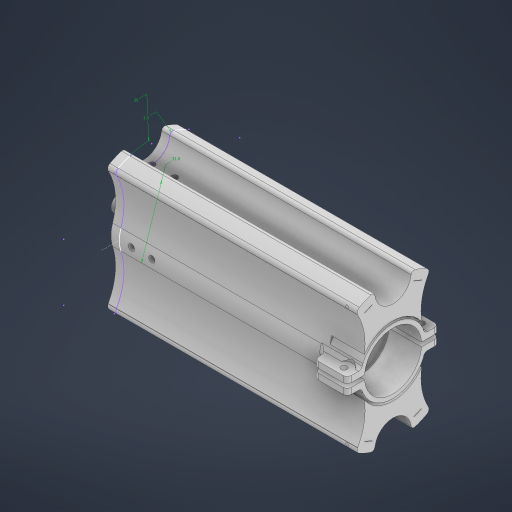
# Autodesk Inventor part: michigandrummy
Saved by Autodesk Inventor 2024.2 (Build 282272000, 272)
## iProperties
Created: 2024-04-03
Part Number: michigandrummy
Material: Generic
Document SubType Name: Modeling
Designer: jerem
Density: 1 g/cm^3
Appearance: Default
Author: jerem
## iProperties of the stored document michigandrummy_3DPrint.ipt
Created: 2024-04-05
Part Number: michigandrummy_3DPrint
Material: Generic
Document SubType Name: Modeling
Designer: jerem
Density: 1 g/cm^3
Appearance: Default
Author: jerem
Autodesk Inventor part; units mm, degrees
ref_plane "YZ Plane" through (0, 0, 0) normal (1, 0, 0) x (0, 1, 0)
ref_plane "XZ Plane" through (0, 0, 0) normal (0, 1, 0) x (-1, 0, 0)
ref_plane "XY Plane" through (0, 0, 0) normal (0, 0, 1) x (1, 0, 0)
sketch "Sketch1" plane through (0, 0, 0) normal (1, 0, 0) x (0, 1, 0)
  arc A0 (1, -13.864) -> (1, 13.864) centre (0, 0) ccw
  line L0 (0, 0) -> (1, 0) construction
  line L1 (1, 13.864) -> (1, 22.3886)
  line L2 (1, 22.3886) -> (4, 22.3886)
  line L3 (4, 22.3886) -> (4, 15.3886)
  line L4 (1, -13.864) -> (1, -22.3886)
  line L5 (1, -22.3886) -> (4, -22.3886)
  line L6 (4, -22.3886) -> (4, -15.3886)
  arc A1 (4, -15.3886) -> (4, 15.3886) centre (0, 0) ccw
  point P0 (4, -15.3886)
  point P1 (4, 15.3886)
  dimension "d0" = 27.8
  dimension "d1" = 1
  dimension "d3" = 3
  dimension "d4" = 2
  dimension "d5" = 1
  dimension "d11" = 7
  constraints: 14 end point, 4 point on circle, 2 centre point, 2 coincident, 2 collinear, 2 horizontal, 2 symmetric about line, 1 perpendicular, 1 vertical
  measures "d0" diameter of A0
  measures "d1" distance of L0.start L0.end
  measures "d3" distance of L1.end L2.end
  measures "d4" radial gap between concentric circles of A0 A1
  measures "d5" distance from line of point (0, 0) L1
  measures "d11" distance of L3.end L2.end
extrude "Extrusion1" add sketch "Sketch1" along normal blind 16
sketch "Sketch2" plane through (0, 4, 22.3886) normal (0, 1, 0) x (1, 0, 0)
  line L0 (0, 7) -> (16, 7) construction
  line L1 (16, 0) -> (16, 8.5247) construction
  line L2 (16, 7) -> (16, 0) construction
  circle A0 centre (11, 3.5) radius 1.5
  line L3 (16, 36.2526) -> (16, 8.5247) projected
  line L4 (16, 22.3886) -> (0, 22.3886)
  circle A1 centre (11, 41.2773) radius 1.5
  line L5 (11, 41.2773) -> (11, 37.7773) construction
  line L6 (0, 37.7773) -> (16, 37.7773) construction
  line L7 (11, 3.5) -> (11, 7) construction
  point P0 (16, 3.5)
  dimension "d8" = 5
  dimension "d9" = 3
  dimension "d10" = 3.5
  constraints: 8 end point, 3 point on line, 2 centre point, 2 midpoint, 1 collinear, 1 horizontal, 1 symmetric about line, 1 vertical, 1 other
  measures "d8" distance of point (16, 3.5) L7.start
  measures "d9" diameter of A0
  measures "d10" distance of L7.start L7.end
extrude "Extrusion2" cut sketch "Sketch2" along normal through all both and the other way through all
mirror "Mirror1" about plane through (0, 0, 0) normal (0, 1, 0) of "Extrusion1", "Extrusion2"
fillet "Fillet1" radius 2 4 edges at (8, 4, 15.3886) (8, -4, 15.3886) (8, 4, -15.3886) (8, -4, -15.3886)
sketch "Sketch3" plane through (0, -4, -22.3886) normal (-1, 0, 0) x (0, 0, 1)
  circle A0 centre (22.3886, 4) radius 13.9
  circle A1 centre (22.3886, 4) radius 15.9
  circle A2 centre (22.3886, 4) radius 4.85
  dimension "d15" = 9.7
  dimension "d19" = 27.8
  dimension "d20" = 2
  constraints: 3 centre point, 3 coincident
  measures "d15" diameter of A2
  measures "d19" diameter of A0
  measures "d20" radial gap between concentric circles of A0 A1
extrude "Extrusion3" add sketch "Sketch3" along normal blind 4.2 contours A0 | A1
sketch "Sketch4" plane through (-4.2, 0, 0) normal (-1, 0, 0) x (0, 0, 1)
  circle A0 centre (0, 0) radius 4.85
  circle A1 centre (0, 0) radius 15.9
  circle A2 centre (0, 0) radius 4.85 projected
  circle A3 centre (0, 0) radius 1.5
  dimension "d18" = 3
  dimension "d21" = 31.8
  constraints: 3 centre point, 2 coincident
  measures "d18" diameter of A3
  measures "d21" diameter of A1
extrude "Extrusion4" add sketch "Sketch4" along normal blind 10 contours A0 | A1
fillet "Fillet2" radius 4 4 edges at (0, -3.1958, 15.5755) (0, 3.1958, 15.5755) (0, -3.1958, -15.5755) (0, 3.1958, -15.5755)
sketch "Sketch5" plane through (-14.2, 0, 0) normal (-1, 0, 0) x (0, 0, 1)
  circle A0 centre (0, 0) radius 1.5 projected
  circle A1 centre (0, 0) radius 2
  circle A2 centre (0, 0) radius 4
  dimension "d25" = 4
  dimension "d26" = 2
  constraints: 2 centre point, 2 coincident
  measures "d25" diameter of A1
  measures "d26" radial gap between concentric circles of A1 A2
extrude "Extrusion5" add sketch "Sketch5" along normal blind 87.8 contours A2
sketch "Sketch6" plane through (0, 0, 0) normal (1, 0, 0) x (0, 1, 0)
  circle A0 centre (0, 0) radius 1.5 construction
  circle A1 centre (0, 0) radius 35 construction
  line L0 (35, 0) -> (25, 0)
  line L1 (31.6536, -14.9349) -> (22.6097, -10.6678)
  arc A2 (31.6536, -14.9349) -> (35, 0) centre (0, 0) ccw construction
  dimension "d29" = 70
  dimension "d30" = 10
  dimension "d31" = 10
  constraints: 4 end point, 4 point on circle, 2 centre point, 1 coincident, 1 concentric, 1 horizontal, 1 line through centre
  measures "d29" diameter of A1
  measures "d30" distance of L0.start L0.end
  measures "d31" distance of L1.start L1.end
sketch "Sketch7" plane through (-102, 0, 0) normal (-1, 0, 0) x (0, 0, 1)
  circle A0 centre (0, 0) radius 15.9
  circle A1 centre (0, 0) radius 1.5 projected
  line L0 (0, 0) -> (24.7477, 0) construction
  line L1 (-24.9082, 0) -> (-15.9, 0)
  line L2 (-1.5, 0) -> (15.9, 0)
  line L3 (17.3493, 28.2476) -> (17.2713, 28.1124)
  line L4 (0.1605, 0) -> (15.9, 0)
  arc A2 (0, 24.1323) -> (8.826, 31.8269) centre (0, 33.0415) ccw
  arc A3 (17.3493, 28.2476) -> (15.119, 4.9221) centre (43.0631, 14.0195) ccw
  arc A4 (0, 24.1323) -> (8.852, 32.0333) centre (0, 33.0415) ccw
  arc A5 (16.481, 30.8768) -> (10.8054, 33.2903) centre (0, 0) ccw
  line L5 (0, 15.9) -> (0, 24.1323)
  line L6 (-17.3493, 28.2476) -> (-17.2713, 28.1124)
  arc A6 (-15.119, 4.9221) -> (-17.3493, 28.2476) centre (-43.0631, 14.0195) ccw
  arc A7 (-8.852, 32.0333) -> (0, 24.1323) centre (0, 33.0415) ccw
  arc A8 (-10.8054, 33.2903) -> (-16.481, 30.8768) centre (0, 0) ccw
  arc A9 (-16.481, 30.8768) -> (-17.2713, 28.1124) centre (-15.5392, 29.1124) ccw
  arc A10 (17.2713, 28.1124) -> (16.481, 30.8768) centre (15.5392, 29.1124) ccw
  arc A11 (-8.852, 32.0333) -> (-10.8054, 33.2903) centre (-10.3423, 31.8636) ccw
  arc A12 (10.8054, 33.2903) -> (8.852, 32.0333) centre (10.3423, 31.8636) ccw
  line L7 (17.3493, -28.2476) -> (17.2713, -28.1124)
  arc A13 (8.826, -31.8269) -> (0, -24.1323) centre (0, -33.0415) ccw
  arc A14 (15.119, -4.9221) -> (17.3493, -28.2476) centre (43.0631, -14.0195) ccw
  arc A15 (8.852, -32.0333) -> (0, -24.1323) centre (0, -33.0415) ccw
  arc A16 (10.8054, -33.2903) -> (16.481, -30.8768) centre (0, 0) ccw
  line L8 (0, -15.9) -> (0, -24.1323)
  arc A17 (-16.481, -30.8768) -> (-10.8054, -33.2903) centre (0, 0) ccw
  arc A18 (-17.3493, -28.2476) -> (-15.119, -4.9221) centre (-43.0631, -14.0195) ccw
  line L9 (-17.3493, -28.2476) -> (-17.2713, -28.1124)
  arc A19 (0, -24.1323) -> (-8.852, -32.0333) centre (0, -33.0415) ccw
  arc A20 (-17.2713, -28.1124) -> (-16.481, -30.8768) centre (-15.5392, -29.1124) ccw
  arc A21 (16.481, -30.8768) -> (17.2713, -28.1124) centre (15.5392, -29.1124) ccw
  arc A22 (-10.8054, -33.2903) -> (-8.852, -32.0333) centre (-10.3423, -31.8636) ccw
  arc A23 (8.852, -32.0333) -> (10.8054, -33.2903) centre (10.3423, -31.8636) ccw
  point P0 (18.2746, 29.8503)
  point P1 (-8.826, 31.8269)
  point P2 (-18.2746, 29.8503)
  point P3 (18.2746, -29.8503)
  point P4 (-8.826, -31.8269)
  point P5 (-18.2746, -29.8503)
  point P6 (8.826, 31.8269)
  point P7 (-15.119, 4.9221)
  point P8 (-15.119, -4.9221)
  point P9 (15.119, -4.9221)
  dimension "d36" = 35
  dimension "d40" = 1.5
  dimension "d41" = 31.8
  constraints: 54 point on circle, 30 symmetric about line, 23 centre point, 20 end point, 9 tangent, 6 point on line, 4 coincident, 2 equal radius, 1 horizontal, 1 horizontal alignment, 15 other
  measures "d36" radius of A5
  measures "d40" radius of A11
  measures "d41" diameter of A0
extrude "Extrusion6" add sketch "Sketch7" against normal up to surface (87.8 mm away)
sketch "Sketch8" plane through (-14.2, 0, 0) normal (1, 0, 0) x (0, 0, -1)
  circle A0 centre (0, 0) radius 35
  circle A1 centre (0, 0) radius 15.9
  arc A2 (-17.3493, -28.2476) -> (-15.119, -4.9221) centre (-43.0631, -14.0195) ccw projected
  arc A3 (15.119, 4.9221) -> (-15.119, 4.9221) centre (0, 0) ccw projected
  arc A4 (17.3493, 28.2476) -> (15.119, 4.9221) centre (43.0631, 14.0195) ccw projected
  line L0 (17.3493, 28.2476) -> (17.2713, 28.1124) projected
  arc A5 (17.2713, 28.1124) -> (16.481, 30.8768) centre (15.5392, 29.1124) ccw projected
  arc A6 (16.481, 30.8768) -> (10.8054, 33.2903) centre (0, 0) ccw projected
  arc A7 (10.8054, 33.2903) -> (8.852, 32.0333) centre (10.3423, 31.8636) ccw projected
  arc A8 (-8.852, 32.0333) -> (8.852, 32.0333) centre (0, 33.0415) ccw projected
  arc A9 (-8.852, 32.0333) -> (-10.8054, 33.2903) centre (-10.3423, 31.8636) ccw projected
  arc A10 (-10.8054, 33.2903) -> (-16.481, 30.8768) centre (0, 0) ccw projected
  arc A11 (-16.481, 30.8768) -> (-17.2713, 28.1124) centre (-15.5392, 29.1124) ccw projected
  line L1 (-17.2713, 28.1124) -> (-17.3493, 28.2476) projected
  arc A12 (-15.119, 4.9221) -> (-17.3493, 28.2476) centre (-43.0631, 14.0195) ccw projected
  arc A13 (-15.119, -4.9221) -> (15.119, -4.9221) centre (0, 0) ccw projected
  arc A14 (-17.3493, -28.2476) -> (-15.119, -4.9221) centre (-43.0631, -14.0195) ccw projected
  line L2 (-17.3493, -28.2476) -> (-17.2713, -28.1124) projected
  arc A15 (-17.2713, -28.1124) -> (-16.481, -30.8768) centre (-15.5392, -29.1124) ccw projected
  arc A16 (-16.481, -30.8768) -> (-10.8054, -33.2903) centre (0, 0) ccw projected
  arc A17 (-10.8054, -33.2903) -> (-8.852, -32.0333) centre (-10.3423, -31.8636) ccw projected
  arc A18 (8.852, -32.0333) -> (-8.852, -32.0333) centre (0, -33.0415) ccw projected
  arc A19 (8.852, -32.0333) -> (10.8054, -33.2903) centre (10.3423, -31.8636) ccw projected
  arc A20 (10.8054, -33.2903) -> (16.481, -30.8768) centre (0, 0) ccw projected
  arc A21 (16.481, -30.8768) -> (17.2713, -28.1124) centre (15.5392, -29.1124) ccw projected
  line L3 (17.2713, -28.1124) -> (17.3493, -28.2476) projected
  arc A22 (15.119, -4.9221) -> (17.3493, -28.2476) centre (43.0631, -14.0195) ccw projected
  point P0 (16.481, 30.8768)
  point P1 (10.8054, 33.2903)
  point P2 (-10.8054, 33.2903)
  point P3 (-16.481, 30.8768)
  point P4 (15.119, 4.9221)
  point P5 (-17.3493, -28.2476)
  point P6 (-16.481, -30.8768)
  point P7 (-10.8054, -33.2903)
  point P8 (10.8054, -33.2903)
  point P9 (16.481, -30.8768)
  point P10 (15.119, -4.9221)
  dimension "d44" = 70
  constraints: 2 coincident, 1 centre point, 2 other
  measures "d44" diameter of A0
extrude "Extrusion7" add sketch "Sketch8" along normal up to surface (30.2 mm away) contours A5 L0 A4 A1 A12 L1 A11 A0 A9 A8 A7 | A0 A19 A18 A17 A15 L2 A2 A1 A22 L3 A21
sketch "Sketch10" plane through (0, 4, 22.3886) normal (0, 1, 0) x (1, 0, 0)
  circle A0 centre (11, 3.5) radius 1.5 projected
  circle A1 centre (11, 41.2773) radius 1.5 projected
  circle A2 centre (11, 3.5) radius 1.5
  circle A3 centre (11, 41.2773) radius 1.5
  point P0 (0, 22.3886)
  point P1 (12.8189, 5.5242)
  point P2 (9.3832, 5.5242)
  point P3 (9.3832, 39.2531)
  point P4 (12.8189, 39.2531)
  point P5 (9.7518, 39.7146)
  point P6 (12.5, 41.2773)
  point P7 (12.3368, 4.9876)
  point P8 (12.5, 3.5)
  constraints: 2 centre point, 2 coincident, 4 other
extrude "Extrusion8" cut sketch "Sketch10" along normal mid plane 147.627
sketch "Sketch12" plane through (16, 0, 0) normal (1, 0, 0) x (0, 0, -1)
  arc A0 (17.3493, 28.2476) -> (15.0262, 5.212) centre (43.0631, 14.0195) ccw projected
  line L0 (17.2713, 28.1124) -> (17.3493, 28.2476) projected
  arc A1 (17.2713, 28.1124) -> (16.481, 30.8768) centre (15.5392, 29.1124) ccw projected
  arc A2 (16.481, 30.8768) -> (10.8054, 33.2903) centre (0, 0) ccw projected
  arc A3 (10.8054, 33.2903) -> (8.852, 32.0333) centre (10.3423, 31.8636) ccw projected
  arc A4 (-8.852, 32.0333) -> (8.852, 32.0333) centre (0, 33.0415) ccw projected
  arc A5 (-8.852, 32.0333) -> (-10.8054, 33.2903) centre (-10.3423, 31.8636) ccw projected
  arc A6 (-10.8054, 33.2903) -> (-16.481, 30.8768) centre (0, 0) ccw projected
  arc A7 (-16.481, 30.8768) -> (-17.2713, 28.1124) centre (-15.5392, 29.1124) ccw projected
  line L1 (-17.3493, 28.2476) -> (-17.2713, 28.1124) projected
  arc A8 (-15.0262, 5.212) -> (-17.3493, 28.2476) centre (-43.0631, 14.0195) ccw projected
  arc A9 (-16.8645, 4) -> (-15.0262, 5.212) centre (-16.8645, 6) ccw projected
  line L2 (-16.8645, 4) -> (-22.3886, 4) projected
  line L3 (-22.3886, 4) -> (-22.3886, 1) projected
  line L4 (-22.3886, 1) -> (-13.864, 1) projected
  arc A10 (13.864, 1) -> (-13.864, 1) centre (0, 0) ccw projected
  line L5 (13.864, 1) -> (22.3886, 1) projected
  line L6 (22.3886, 1) -> (22.3886, 4) projected
  line L7 (22.3886, 4) -> (16.8645, 4) projected
  arc A11 (15.0262, 5.212) -> (16.8645, 4) centre (16.8645, 6) ccw projected
  line L8 (-13.9332, 27.3327) -> (-10.2755, 28.8831)
  line L9 (-10.2755, 28.8831) -> (-10.1975, 28.6989)
  line L10 (-10.1975, 28.6989) -> (-13.8551, 27.1485)
  line L11 (-13.8551, 27.1485) -> (-13.9332, 27.3327)
  line L12 (-14.2092, 31.9859) -> (-14.2092, 31.9859)
  point P0 (-17.3103, 28.18)
  point P1 (-13.8941, 27.2406)
  point P2 (-10.2365, 28.791)
  point P3 (-12.1043, 28.1079)
  dimension "d63" = 0.2
  constraints: 10 end point, 4 midpoint, 3 perpendicular, 2 point on circle, 1 tangent
  measures "d63" distance from line of L10 point (-12.104, 28.108)
extrude "Extrusion10" cut sketch "Sketch12" against normal through all contours L8 L9 L10 L11
mirror "Mirror4" about plane through (0, 0, 0) normal (0, 1, 0) of "Extrusion10"
mirror "Mirror5" about plane through (0, 0, 0) normal (0, 0, 1) of "Extrusion10", "Mirror4"
extrude "Extrusion12" add sketch "Sketch7" along normal blind 4
sketch "Sketch13" plane through (-102, 0, 0) normal (-1, 0, 0) x (0, 0, 1)
  circle A0 centre (0, 0) radius 3.925
  circle A1 centre (0, 0) radius 1.5 projected
  circle A2 centre (0, 0) radius 1.5
  dimension "d64" = 7.85
  dimension "d65" = 3
  constraints: 2 centre point, 2 coincident
  measures "d64" diameter of A0
  measures "d65" diameter of A2
extrude "Extrusion11" add sketch "Sketch13" along normal blind 12 from surface at 4
sketch "Sketch14" plane through (-106, 0, 0) normal (-1, 0, 0) x (0, 0, 1)
  circle A0 centre (0, 0) radius 4.445
  circle A1 centre (0, 0) radius 2
  dimension "d70" = 8.89
  constraints: 2 centre point, 2 coincident
  measures "d70" diameter of A0
extrude "Extrusion13" add sketch "Sketch14" along normal blind 2 contours A0 | A1
sketch "Sketch15" plane through (16, 0, 0) normal (1, 0, 0) x (0, 0, -1)
  circle A0 centre (0, 0) radius 14
  dimension "d73" = 28
  constraints: 1 centre point, 1 coincident
  measures "d73" diameter of A0
extrude "Extrusion14" cut sketch "Sketch15" against normal up to surface (16 mm away)
sketch "Sketch16" plane through (0, 4, 22.3886) normal (0, 1, 0) x (1, 0, 0)
  circle A0 centre (11, 3.5) radius 1.5 projected
  circle A1 centre (11, 3.5) radius 4
  point P0 (0, 22.3886)
  dimension "d76" = 8
  constraints: 1 centre point, 1 coincident
  measures "d76" diameter of A1
extrude "Extrusion15" cut sketch "Sketch16" along normal blind 10
mirror "Mirror6" about plane through (0, 0, 0) normal (0, 1, 0) of "Extrusion15"
mirror "Mirror7" about plane through (0, 0, 0) normal (0, 0, 1) of "Extrusion15", "Mirror6"
sketch "Sketch17" plane through (16, 0, 0) normal (1, 0, 0) x (0, 0, -1)
  circle A0 centre (0, 0) radius 4.85 projected
  circle A1 centre (0, 0) radius 16
  circle A2 centre (0, 0) radius 1.5 projected
  circle A3 centre (0, 0) radius 17
  arc A4 (13.9642, 1) -> (-13.9642, 1) centre (0, 0) ccw projected
  line L0 (13.9642, 1) -> (22.3886, 1) projected
  line L1 (22.3886, 1) -> (22.3886, 4) projected
  line L2 (22.3886, 4) -> (16.8645, 4) projected
  arc A5 (15.0262, 5.212) -> (16.8645, 4) centre (16.8645, 6) ccw projected
  arc A6 (17.3493, 28.2476) -> (15.0262, 5.212) centre (43.0631, 14.0195) ccw projected
  line L3 (17.2713, 28.1124) -> (17.3493, 28.2476) projected
  arc A7 (17.2713, 28.1124) -> (16.481, 30.8768) centre (15.5392, 29.1124) ccw projected
  arc A8 (16.481, 30.8768) -> (10.8054, 33.2903) centre (0, 0) ccw projected
  arc A9 (10.8054, 33.2903) -> (8.852, 32.0333) centre (10.3423, 31.8636) ccw projected
  arc A10 (-8.852, 32.0333) -> (8.852, 32.0333) centre (0, 33.0415) ccw projected
  arc A11 (-8.852, 32.0333) -> (-10.8054, 33.2903) centre (-10.3423, 31.8636) ccw projected
  arc A12 (-10.8054, 33.2903) -> (-16.481, 30.8768) centre (0, 0) ccw projected
  arc A13 (-16.481, 30.8768) -> (-17.2713, 28.1124) centre (-15.5392, 29.1124) ccw projected
  line L4 (-17.3493, 28.2476) -> (-17.2713, 28.1124) projected
  arc A14 (-15.0262, 5.212) -> (-17.3493, 28.2476) centre (-43.0631, 14.0195) ccw projected
  arc A15 (-16.8645, 4) -> (-15.0262, 5.212) centre (-16.8645, 6) ccw projected
  line L5 (-16.8645, 4) -> (-22.3886, 4) projected
  line L6 (-22.3886, 4) -> (-22.3886, 1) projected
  line L7 (-22.3886, 1) -> (-13.9642, 1) projected
  line L8 (13.9332, 27.3327) -> (13.8551, 27.1485) projected
  line L9 (13.8551, 27.1485) -> (10.1975, 28.6989) projected
  line L10 (10.1975, 28.6989) -> (10.2755, 28.8831) projected
  line L11 (10.2755, 28.8831) -> (13.9332, 27.3327) projected
  line L12 (-10.2755, 28.8831) -> (-10.1975, 28.6989) projected
  line L13 (-10.1975, 28.6989) -> (-13.8551, 27.1485) projected
  line L14 (-13.8551, 27.1485) -> (-13.9332, 27.3327) projected
  line L15 (-13.9332, 27.3327) -> (-10.2755, 28.8831) projected
  arc A16 (-13.9642, -1) -> (13.9642, -1) centre (0, 0) ccw projected
  line L16 (-22.3886, -1) -> (-13.9642, -1) projected
  line L17 (-22.3886, -4) -> (-22.3886, -1) projected
  line L18 (-16.8645, -4) -> (-22.3886, -4) projected
  arc A17 (-15.0262, -5.212) -> (-16.8645, -4) centre (-16.8645, -6) ccw projected
  arc A18 (-17.3493, -28.2476) -> (-15.0262, -5.212) centre (-43.0631, -14.0195) ccw projected
  line L19 (-17.2713, -28.1124) -> (-17.3493, -28.2476) projected
  arc A19 (-17.2713, -28.1124) -> (-16.481, -30.8768) centre (-15.5392, -29.1124) ccw projected
  arc A20 (-16.481, -30.8768) -> (-10.8054, -33.2903) centre (0, 0) ccw projected
  arc A21 (-10.8054, -33.2903) -> (-8.852, -32.0333) centre (-10.3423, -31.8636) ccw projected
  arc A22 (8.852, -32.0333) -> (-8.852, -32.0333) centre (0, -33.0415) ccw projected
  arc A23 (8.852, -32.0333) -> (10.8054, -33.2903) centre (10.3423, -31.8636) ccw projected
  arc A24 (10.8054, -33.2903) -> (16.481, -30.8768) centre (0, 0) ccw projected
  arc A25 (16.481, -30.8768) -> (17.2713, -28.1124) centre (15.5392, -29.1124) ccw projected
  line L20 (17.3493, -28.2476) -> (17.2713, -28.1124) projected
  arc A26 (15.0262, -5.212) -> (17.3493, -28.2476) centre (43.0631, -14.0195) ccw projected
  arc A27 (16.8645, -4) -> (15.0262, -5.212) centre (16.8645, -6) ccw projected
  line L21 (22.3886, -4) -> (16.8645, -4) projected
  line L22 (22.3886, -1) -> (22.3886, -4) projected
  line L23 (13.9642, -1) -> (22.3886, -1) projected
  line L24 (-13.9332, -27.3327) -> (-13.8551, -27.1485) projected
  line L25 (-13.8551, -27.1485) -> (-10.1975, -28.6989) projected
  line L26 (-10.1975, -28.6989) -> (-10.2755, -28.8831) projected
  line L27 (-10.2755, -28.8831) -> (-13.9332, -27.3327) projected
  line L28 (13.8551, -27.1485) -> (13.9332, -27.3327) projected
  line L29 (13.9332, -27.3327) -> (10.2755, -28.8831) projected
  line L30 (10.2755, -28.8831) -> (10.1975, -28.6989) projected
  line L31 (10.1975, -28.6989) -> (13.8551, -27.1485) projected
  point P0 (14.0038, -9.6381)
  point P1 (14.7072, -6.3007)
  point P2 (-14.7072, -6.3007)
  point P3 (-14.0038, -9.6381)
  point P4 (-14.0038, 9.6381)
  point P5 (-14.7072, 6.3007)
  point P6 (14.7072, 6.3007)
  point P7 (14.0038, 9.6381)
  dimension "d79" = 32
  dimension "d80" = 34
  constraints: 2 centre point, 2 coincident
  measures "d79" diameter of A1
  measures "d80" diameter of A3
extrude "Extrusion16" cut sketch "Sketch17" against normal up to surface (16 mm away) contours A1 A14 A3 A6 | A26 A3 A18 A1
extrude "Extrusion17" cut sketch "Sketch4" along normal blind 20 contours A3
sketch "Sketch18" plane through (0, 0, 0) normal (0, 0, 1) x (1, 0, 0)
  line L0 (-106, 4.9221) -> (-106, -4.9221) construction
  line L1 (-106, 0) -> (-96, 0) construction
  circle A0 centre (-96, 0) radius 1.5
  line L2 (-4, 4.9221) -> (-106, 4.9221) projected
  line L3 (-96, 0) -> (-86, 0)
  circle A1 centre (-86, 0) radius 1.5
  point P0 (0, 0)
  dimension "d85" = 10
  dimension "d86" = 3
  dimension "d96" = 10
  dimension "d97" = 3
  constraints: 4 end point, 2 centre point, 2 coincident, 2 horizontal, 1 midpoint
  measures "d85" distance of L1.start L1.end
  measures "d86" diameter of A0
  measures "d96" distance of L3.start L3.end
  measures "d97" diameter of A1
extrude "Extrusion18" cut sketch "Sketch18" along normal through all both and the other way through all
extrude "Extrusion19" cut sketch "Sketch7" along normal up to surface (16 mm away) contours L2 A1 | A1 L2
sketch "Sketch19" plane through (0, 0, 0) normal (0, 1, 0) x (-1, 0, 0)
  line L0 (106, 8.852) -> (106, -8.852) projected
  line L1 (106, 0) -> (91, 0)
  circle A0 centre (91, 0) radius 1.5
  line L2 (94.5, -1.5) -> (87.5, -1.5) projected
  circle A1 centre (102, 0) radius 1.5
  point P0 (0, 0)
  dimension "d91" = 15
  dimension "d94" = 3
  constraints: 2 centre point, 2 end point, 1 coincident, 1 horizontal, 1 midpoint, 1 point on line, 1 tangent
  measures "d91" distance of L1.start L1.end
  measures "d94" diameter of A1
extrude "Extrusion20" cut sketch "Sketch19" along normal through all both and the other way through all
chamfer "Chamfer1" distance 2 angle 45 1 edges at (-106, 0, -4.445)
fillet "Fillet3" radius 2 8 edges at (0, 2.5, 22.3886) (0, -2.5, 22.3886) (0, -2.5, -22.3886) (0, 2.5, -22.3886) (16, -2.5, -22.3886) (16, 2.5, -22.3886) (16, -2.5, 22.3886) (16, 2.5, 22.3886)
sketch "Sketch11" plane through (16, 0, 0) normal (1, 0, 0) x (0, 0, -1)
  line L0 (-15.514, 28.2777) -> (-16.3831, 27.7832)
  line L1 (-16.3831, 27.7832) -> (-16.814, 29.5515)
  line L2 (-16.814, 29.5515) -> (-15.514, 28.2777)
  arc A0 (17.3493, 28.2476) -> (15.0262, 5.212) centre (43.0631, 14.0195) ccw projected
  line L3 (17.2713, 28.1124) -> (17.3493, 28.2476) projected
  arc A1 (17.2713, 28.1124) -> (16.481, 30.8768) centre (15.5392, 29.1124) ccw projected
  arc A2 (16.481, 30.8768) -> (10.8054, 33.2903) centre (0, 0) ccw projected
  arc A3 (10.8054, 33.2903) -> (8.852, 32.0333) centre (10.3423, 31.8636) ccw projected
  arc A4 (-8.852, 32.0333) -> (8.852, 32.0333) centre (0, 33.0415) ccw projected
  arc A5 (-8.852, 32.0333) -> (-10.8054, 33.2903) centre (-10.3423, 31.8636) ccw projected
  arc A6 (-10.8054, 33.2903) -> (-16.481, 30.8768) centre (0, 0) ccw projected
  arc A7 (-16.481, 30.8768) -> (-17.2713, 28.1124) centre (-15.5392, 29.1124) ccw projected
  line L4 (-17.3493, 28.2476) -> (-17.2713, 28.1124) projected
  arc A8 (-15.0262, 5.212) -> (-17.3493, 28.2476) centre (-43.0631, 14.0195) ccw projected
  arc A9 (-16.8645, 4) -> (-15.0262, 5.212) centre (-16.8645, 6) ccw projected
  line L5 (-16.8645, 4) -> (-20.3886, 4) projected
  line L6 (-20.3886, 4) -> (-20.3886, 1) projected
  line L7 (-20.3886, 1) -> (-13.864, 1) projected
  arc A10 (13.864, 1) -> (-13.864, 1) centre (0, 0) ccw projected
  line L8 (13.864, 1) -> (20.3886, 1) projected
  line L9 (20.3886, 1) -> (20.3886, 4) projected
  line L10 (20.3886, 4) -> (16.8645, 4) projected
  arc A11 (15.0262, 5.212) -> (16.8645, 4) centre (16.8645, 6) ccw projected
  circle A12 centre (0, 0) radius 1.5 construction
  circle A13 centre (0, 0) radius 35 construction
  line L11 (-16.814, 29.5515) -> (-15.9485, 28.0305) construction
  line L12 (-15.2443, 30.391) -> (-14.4597, 28.8267) construction
  line L13 (-14.9066, 28.6025) -> (-15.2443, 30.391)
  line L14 (-15.2443, 30.391) -> (-14.0128, 29.0509)
  line L15 (-14.0128, 29.0509) -> (-14.9066, 28.6025)
  line L16 (-13.6329, 31.1471) -> (-12.9312, 29.544) construction
  line L17 (-13.3892, 29.3435) -> (-13.6329, 31.1471)
  line L18 (-13.6329, 31.1471) -> (-12.4732, 29.7445)
  line L19 (-12.4732, 29.7445) -> (-13.3892, 29.3435)
  line L20 (-11.9841, 31.8179) -> (-11.3673, 30.1803) construction
  line L21 (-11.8352, 30.004) -> (-11.9841, 31.8179)
  line L22 (-11.9841, 31.8179) -> (-10.8994, 30.3565)
  line L23 (-10.8994, 30.3565) -> (-11.8352, 30.004)
  line L24 (-10.3024, 32.4015) -> (-9.7722, 30.7338) construction
  line L25 (-10.2487, 30.5823) -> (-10.3024, 32.4015)
  line L26 (-10.3024, 32.4015) -> (-9.2957, 30.8853)
  line L27 (-9.2957, 30.8853) -> (-10.2487, 30.5823)
  line L28 (-16.3831, 27.7832) -> (-16.9459, 27.4928) construction
  line L29 (-9.2957, 30.8853) -> (-8.6788, 31.0284) construction
  arc A14 (-8.852, 32.0333) -> (8.852, 32.0333) centre (0, 33.0415) ccw construction
  dimension "d49" = 34
  dimension "d50" = 1.75
  dimension "d51" = 1
  dimension "d54" = 12
  constraints: 44 end point, 3 line through centre, 2 equal length, 2 point on circle, 1 centre point, 1 coincident, 1 concentric, 1 midpoint, 33 other
  measures "d49" distance of A13.centre L1.end
  measures "d50" distance of L1.end L11.end
  measures "d51" distance of L0.start L0.end
body "Solid1"
